Autodesk Inventor part; units mm, degrees
(part 2 of 2)
extrude "Выдавливание35" cut sketch "Эскиз14" against normal blind 4 from surface at -22.8 contours A22 L145 A21 | L145 A21 A22 | A21 L145 | L145 A21
extrude "Выдавливание36" cut sketch "Эскиз14" against normal blind 5.4 contours L163 L145 A2 L161 A23 | L163 L24 A2 L145 | L161 A2 L159 A23 | A23 L123 L144 L162 | L145 A1 L161 A2 | A2 L24 L163 L13 A1 L145 | L161 A1 L159 A2 | L159 A2 L145 L132 A23 | L144 L123 L29 L28 A12 L105 L106 L107 L108 L164 L23 A3 L154 L155 L156 L162 | A23 L114 A12 L29 L123 | L145 A22 A1 | A1 L13 L163 A4 L164 L14 L145 A22 | L159 A1 L145 A2 | L132 L27 A9 L121 A23 | L121 A9 L92 A23 | A3 L156 A0 L162 | A23 L104 A12 L114 | A22 L145 A21 | L145 A21 A22 | L163 L164 A4 | L145 A1 L14 L164 L23 A2 | A2 L23 L164 L108 L109 L90 L91 A9 L28 L27 L132 L145 | L121 L76 A23 L92 A9 | A9 L27 L121 | A23 L76 L27 | L27 A7 L28 L164 A23 | A23 L164 L28 A8 L29 | L29 L62 A23 | A23 L62 L114 A12 L104 | L29 A12 L28 | L156 L155 L154 A3 L21 L20 L19 | A3 L19 A0 L156 | A0 L156 L157 L154 L14 L164 A4 L162 | L114 L29 A12 | A21 L145 | L145 A21 | A4 L164 L162 | L27 L28 A9 | A9 L28 A7 L27 | A8 L28 A12 L29 | A3 L21 A0 L19 | L19 L20 L21 A3 | A0 L22 L154 L157 L156 | L164 L14 A0 L154 A3 L23 | A9 L91 L90 L109 L108 L164 L28 L85 L83 L84 | L84 L83 L85 L28 | L164 L108 L107 L106 L105 A12 L28 L80 L81 L82 | L28 L82 L81 L80 | A0 L22 | A3 L154 A0 L21
ref_plane "РабПлоскость8" through (-36.9, -3.3675, 44.2) normal (0, 0, -1) x (-1, 0, 0)
sketch "Эскиз18" plane through (-36.9, -3.3675, 44.2) normal (0, 0, -1) x (-1, 0, 0)
  line L0 (41.6, 3.3675) -> (41.6, 13.5675) projected
  line L1 (41.6, 13.5675) -> (41.6, 5.1675)
  line L2 (41.6, 5.1675) -> (20.65, 5.1675) construction
  line L3 (20.65, 5.1675) -> (20.65, -10.2325) construction
  line L4 (15.55, 0.0675) -> (25.75, 0.0675)
  line L5 (25.75, 0.0675) -> (25.75, -5.1325)
  line L6 (25.75, -5.1325) -> (15.55, -5.1325)
  line L7 (15.55, -5.1325) -> (15.55, 0.0675)
  line L8 (15.55, 0.0675) -> (25.75, -5.1325) construction
  line L9 (25.75, 0.0675) -> (15.55, -5.1325) construction
  point P0 (-36.9, 3.3675)
  point P1 (20.65, -2.5325)
  dimension "d339" = 8.4
  dimension "d340" = 20.95
  dimension "d341" = 15.4
  dimension "d342" = 10.2
  dimension "d343" = 5.2
  constraints: 18 end point, 3 midpoint, 2 horizontal, 2 parallel, 2 perpendicular, 1 point on line
  measures "d339" distance of L0.end L1.end
  measures "d340" distance of L1.end L2.end
  measures "d341" distance of L2.end L3.end
  measures "d342" distance of L5.end L6.end
  measures "d343" distance of L4.end L5.end
extrude "Выдавливание37" cut sketch "Эскиз18" against normal blind 2.1 from surface at -15.2
extrude "Выдавливание38" cut sketch "Эскиз18" along normal blind 2.1 from surface at 15.2
sketch "Эскиз19" plane through (-78.5, 10.2, 0) normal (0, 1, 0) x (1, 0, 0)
  line L0 (0, 0) -> (0, -88.4) projected
  line L1 (0, -88.4) -> (157, -88.4) projected
  line L2 (0, 0) -> (157, 0)
  line L3 (157, 0) -> (157, -88.4)
  line L4 (157, -88.4) -> (0, -88.4)
  line L5 (0, -88.4) -> (0, 0)
  line L6 (157, 0) -> (157, -88.4) projected
  line L7 (157, -44.2) -> (0, -44.2) construction
  line L8 (78.5, -88.4) -> (78.5, 0) construction
  line L9 (1.6, -1.6) -> (155.4, -1.6)
  line L10 (155.4, -1.6) -> (155.4, -86.8)
  line L11 (155.4, -86.8) -> (1.6, -86.8)
  line L12 (1.6, -86.8) -> (1.6, -1.6)
  line L13 (1.6, -1.6) -> (155.4, -86.8) construction
  line L14 (155.4, -1.6) -> (1.6, -86.8) construction
  point P0 (78.5, -44.2)
  dimension "d348" = 157
  dimension "d349" = 88.4
  dimension "d350" = 153.8
  dimension "d351" = 85.2
  constraints: 24 end point, 6 midpoint, 4 parallel, 2 horizontal, 2 perpendicular, 1 vertical
  measures "d348" distance of L1.end L4.end
  measures "d349" distance of L2.end L1.end
  measures "d350" distance of L10.end L11.end
  measures "d351" distance of L9.end L10.end
extrude "Выдавливание39" add sketch "Эскиз19" along normal blind 20
sketch "Эскиз20" plane through (0, 0, 0) normal (0, 0, -1) x (-1, 0, 0)
  line L0 (-78.5, 0) -> (-78.5, 30.2) projected
  line L1 (-78.5, 30.2) -> (78.5, 30.2)
  line L2 (78.5, 30.2) -> (78.5, 30.2)
  line L3 (78.5, 30.2) -> (-78.5, 30.2)
  line L4 (-78.5, 30.2) -> (-78.5, 30.2)
  line L5 (0, 30.2) -> (0, 10.2) construction
  line L6 (0, 10.2) -> (-5, 10.2)
  line L7 (-5, 10.2) -> (-28.8351, 30.2)
  line L8 (-76.9, 30.2) -> (76.9, 30.2) projected
  line L9 (-5, 10.2) -> (26.1145, 10.2) construction
  line L10 (0, 10.2) -> (5, 10.2)
  line L11 (5, 10.2) -> (28.8351, 30.2)
  point P0 (0, 0)
  point P1 (-28.8351, 30.2)
  point P2 (-28.8351, 30.2)
  point P3 (28.8351, 30.2)
  point P4 (28.8351, 30.2)
  dimension "d354" = 157
  dimension "d355" = 0
  dimension "d356" = 20
  dimension "d357" = 5
  dimension "d363" = 140
  constraints: 20 end point, 3 equal length, 3 horizontal, 2 symmetric about line, 1 midpoint, 1 perpendicular, 1 point on line, 1 vertical
  measures "d354" distance of L2.end L3.end
  measures "d355" distance of L1.end L2.end
  measures "d356" distance of L5.start L5.end
  measures "d357" distance of L5.end L6.end
  measures "d363" angle of L9 L7
extrude "Выдавливание40" add sketch "Эскиз20" along normal blind 22.5
extrude "Выдавливание41" add sketch "Эскиз20" against normal blind 22.5 from surface at -88.4
extrude "Выдавливание42" cut sketch "Эскиз10" along normal blind 2 from surface at -6 contours L67 L24 L68 L7 | L7 L54 L9 L50 | L9 L69 L26 L66 | L24 L72 L7 L70 | L7 L63 L9 L58 | L71 L9 L73 L26
